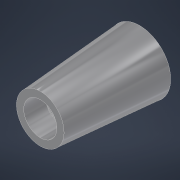
# Autodesk Inventor part: P023-Cage_arbre
Saved by Autodesk Inventor 2021.3 (Build 253353000, 353)
## iProperties
Created: 2022-06-06
Part Number: P023-Cage_arbre
Material: Aluminium
Document SubType Name: Modeling
Designer: Rémi Heredero
Density: 2.7 g/cm^3
Appearance: Aluminum - Dark
Author: Rémi Heredero
Autodesk Inventor part; units mm, degrees
ref_plane "YZ Plane" through (0, 0, 0) normal (1, 0, 0) x (0, 1, 0)
ref_plane "XZ Plane" through (0, 0, 0) normal (0, 1, 0) x (-1, 0, 0)
ref_plane "XY Plane" through (0, 0, 0) normal (0, 0, 1) x (1, 0, 0)
sketch "Sketch3" plane through (0, 0, 0) normal (1, 0, 0) x (0, 1, 0)
  line L0 (-40, 16.5) -> (-40, 11.5)
  line L1 (-40, 11.5) -> (-25, 11.5)
  line L2 (-25, 11.5) -> (-25, 11)
  line L3 (-25, 11) -> (25, 11)
  line L4 (25, 11) -> (25, 11.5)
  line L5 (25, 11.5) -> (29, 11.5)
  line L6 (29, 21.5) -> (-40, 16.5)
  line L7 (-53.8, 0) -> (42.8, 0) projected
  line L8 (29, 11.5) -> (29, 21.5)
  point P0 (0, 0)
  point P1 (0, 11)
  dimension "d1" = 4
  dimension "d2" = 50
  dimension "d6" = 23
  dimension "d7" = 22
  dimension "d8" = 15
  dimension "d9" = 5
  dimension "d10" = 10
  constraints: 16 end point, 4 perpendicular, 2 point on line, 2 vertical, 1 midpoint, 1 vertical alignment
  measures "d1" distance of L4.end L5.end
  measures "d2" distance of L2.end L3.end
  measures "d6" diameter of L1 L7
  measures "d7" diameter of L3 L7
  measures "d8" distance of L0.end L1.end
  measures "d9" distance of L0.start L0.end
  measures "d10" distance of L5.end L6.start
revolve "Revolution1" add sketch "Sketch3" angle 360 about axis through (0, -10, 0) along (0, 1, 0)
sketch "Sketch4" plane through (0, 29, 0) normal (0, 1, 0) x (1, 0, 0)
  circle A0 centre (0, 0) radius 11.5 construction
  circle A1 centre (0, 0) radius 21.5 construction
  circle A2 centre (0, 0) radius 18.1667 construction
  circle A3 centre (0, 0) radius 15
  circle A4 centre (0, 0) radius 16
  dimension "d11" = 23
  dimension "d12" = 43
  dimension "d13" = 36.3333
  dimension "d14" = 30
  dimension "d15" = 1
  constraints: 3 centre point, 3 coincident
  measures "d11" diameter of A0
  measures "d12" diameter of A1
  measures "d13" diameter of A2
  measures "d14" diameter of A3
  measures "d15" radial gap between concentric circles of A4 A3
extrude "Extrusion1" cut sketch "Sketch4" against normal blind 1
equation "\"d13\" = 0.333333 * d11 + 0.666667 * d12"
body "Solid1"
